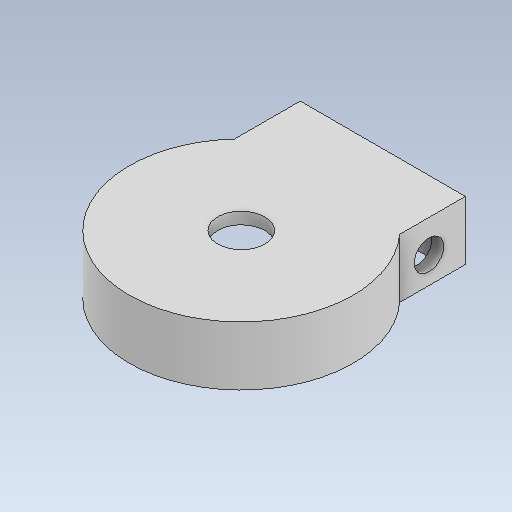
# Autodesk Inventor part: baseSupport
Saved by Autodesk Inventor 2021.2 (Build 252289000, 289)
## iProperties
Created: 2020-11-17
Part Number: baseSupport
Material: Generic
Document SubType Name: Modeling
Designer: robst
Density: 1 g/cm^3
Appearance: Default
Mass: 146.387 g
Surface Area: 500.331 cm^2
Volume: 146.387 cm^3
Author: robst
Autodesk Inventor part; units mm, degrees
ref_plane "YZ Plane" through (0, 0, 0) normal (1, 0, 0) x (0, 1, 0)
ref_plane "XZ Plane" through (0, 0, 0) normal (0, 1, 0) x (-1, 0, 0)
ref_plane "XY Plane" through (0, 0, 0) normal (0, 0, 1) x (1, 0, 0)
sketch "Sketch1" plane through (0, 0, 0) normal (0, 1, 0) x (-1, 0, 0)
  arc A0 (38.1, -38.2321) -> (-38.1, -38.2321) centre (0, 0) ccw
  line L0 (0, 0) -> (0, -72.7817) construction
  line L1 (-38.1, -38.2321) -> (-38.1, -69.85)
  line L2 (-38.1, -69.85) -> (0, -69.85)
  line L3 (0, -69.85) -> (38.1, -69.85)
  line L4 (38.1, -69.85) -> (38.1, -38.2321)
  dimension "d0" = 107.95
  dimension "d6" = 69.85
  dimension "d7" = 38.1
  constraints: 10 end point, 2 perpendicular, 2 point on circle, 2 vertical, 1 centre point, 1 coincident, 1 collinear, 1 horizontal, 1 point on line
  measures "d0" diameter of A0
  measures "d6" distance from line of L2 point (0, 0)
  measures "d7" distance between parallel lines of L1 L0
extrude "Extrusion1" add sketch "Sketch1" along normal blind 6.35
sketch "Sketch3" plane through (0, 0, 0) normal (0, -1, 0) x (1, 0, 0)
  arc A0 (38.1, -38.2321) -> (-38.1, -38.2321) centre (0, 0) ccw projected
  line L0 (38.1, -38.2321) -> (38.1, -69.85) projected
  line L1 (38.1, -69.85) -> (-38.1, -69.85) projected
  line L2 (-38.1, -69.85) -> (-38.1, -38.2321) projected
  arc A1 (38.1, -38.2321) -> (-38.1, -38.2321) centre (0, 0) ccw
  line L3 (38.1, -38.2321) -> (38.1, -69.85) projected
  line L4 (38.1, -38.2321) -> (38.1, -69.85)
  line L5 (38.1, -69.85) -> (-38.1, -69.85)
  line L6 (-38.1, -69.85) -> (-38.1, -38.2321) projected
  line L7 (-38.1, -69.85) -> (-38.1, -38.2321)
  arc A2 (44.45, -40.7836) -> (-44.45, -40.7836) centre (0, 0) ccw
  line L8 (44.45, -40.7836) -> (44.45, -76.2)
  line L9 (44.45, -76.2) -> (-44.45, -76.2)
  line L10 (-44.45, -76.2) -> (-44.45, -40.7836)
  dimension "d8" = 6.35
  dimension "d9" = 6.35
  dimension "d10" = 6.35
  dimension "d11" = 6.35
  constraints: 12 end point, 4 point on circle, 2 centre point, 2 coincident, 2 collinear, 2 perpendicular, 2 vertical, 1 concentric
  measures "d8" radial gap between concentric circles of A2 A0
  measures "d9" distance between parallel lines of L8 L0
  measures "d10" distance between parallel lines of L10 L2
  measures "d11" distance between parallel lines of L9 L1
extrude "Extrusion3" add sketch "Sketch3" along normal blind 25.4
extrude "Extrusion4" add sketch "Sketch3" against normal blind 6.35
sketch "Sketch4" plane through (44.45, -25.4, -40.7836) normal (1, 0, 0) x (0, 0, -1)
  line L0 (20.7014, 17.1105) -> (20.7014, 11.6112) projected
  line L1 (10.9224, 11.4645) -> (10.9224, 17.1105) projected
  line L2 (15.6849, 8.7149) -> (10.9224, 11.4645) projected
  line L3 (20.7014, 11.6112) -> (15.6849, 8.7149) projected
  line L4 (15.8119, 19.9334) -> (20.7014, 17.1105) projected
  line L5 (10.9224, 17.1105) -> (15.8119, 19.9334) projected
  line L6 (10.9224, 17.1105) -> (20.7014, 11.6112) construction
  line L7 (10.9224, 11.4645) -> (20.7014, 17.1105) construction
  circle A0 centre (15.8119, 14.2875) radius 7.9375
  line L8 (20.5744, 17.0371) -> (20.5744, 11.5379)
  line L9 (20.5744, 11.5379) -> (15.8119, 8.7882)
  line L10 (15.8119, 8.7882) -> (11.0494, 11.5379)
  line L11 (11.0494, 11.5379) -> (11.0494, 17.0371)
  line L12 (11.0494, 17.0371) -> (15.8119, 19.7868)
  line L13 (15.8119, 19.7868) -> (20.5744, 17.0371)
  point P0 (-40.7836, 25.4)
  dimension "d20" = 15.875
  dimension "d21" = 9.525
  constraints: 16 end point, 1 centre point, 1 coincident, 1 midpoint, 1 parallel, 13 other
  measures "d20" diameter of A0
  measures "d21" distance between parallel lines of L9 L12
extrude "Extrusion6" cut sketch "Sketch4" against normal up to surface (6.35 mm away) contours L0 L3 L8 L13 L12 L11 L10 L2 L1 L5 L4 | L3 L10 L11 L12 L13 L8 | A0
mirror "Mirror1" about plane through (0, 0, 0) normal (1, 0, 0) of "Extrusion6"
sketch "Sketch5" plane through (0, 6.35, 0) normal (0, 1, 0) x (1, 0, 0)
  circle A0 centre (0, 0) radius 12.7
  dimension "d24" = 25.4
  constraints: 1 centre point, 1 coincident
  measures "d24" diameter of A0
extrude "Extrusion7" cut sketch "Sketch5" against normal through all
equation "\"d0\" = exteriorDiameter"
equation "\"exteriorDiameter\" = 107.95"
body "Solid1"
